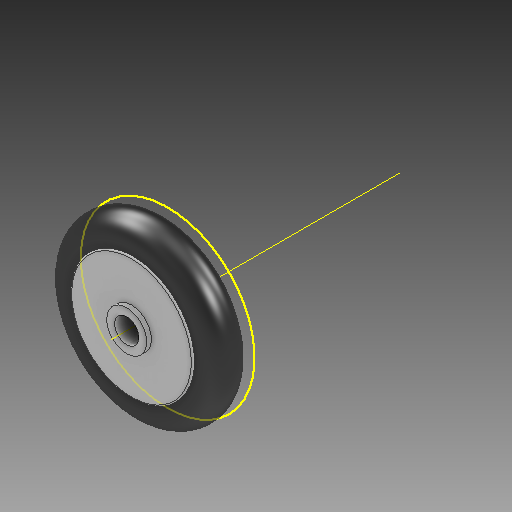
# Autodesk Inventor part: sub_wheel
Saved by Autodesk Inventor 2020 (Build 240168000, 168)
## iProperties
Created: 2024-10-05
Part Number: sub_wheel
Material: Типовые
Document SubType Name: Modeling
Designer: Ivan
Density: 1 g/cm^3
Appearance: По умолчанию
Mass: 0.056422 g
Surface Area: 1.13235 cm^2
Volume: 0.056422 cm^3
Author: Ivan
Autodesk Inventor part; units mm, degrees
ref_plane "YZ Plane" through (0, 0, 0) normal (1, 0, 0) x (0, 1, 0)
ref_plane "XZ Plane" through (0, 0, 0) normal (0, 1, 0) x (-1, 0, 0)
ref_plane "XY Plane" through (0, 0, 0) normal (0, 0, 1) x (1, 0, 0)
sketch "Эскиз1" plane through (0, 0, 0) normal (1, 0, 0) x (0, 1, 0)
  line L0 (0, 0.95) -> (0, -0.95)
  line L1 (0, 0) -> (5, 0) construction
  arc A0 (2.5342, 0.6562) -> (2.5342, -0.6562) centre (2.8973, 0) ccw
  line L2 (2.8973, 0.75) -> (2.8973, -0.75)
  line L3 (2.51, 0.75) -> (0, 0.75)
  line L4 (2.51, -0.75) -> (0, -0.75)
  arc A1 (2.5342, 0.6562) -> (2.51, 0.75) centre (2.51, 0.7) ccw
  arc A2 (2.51, -0.75) -> (2.5342, -0.6562) centre (2.51, -0.7) ccw
  line L5 (0.8367, 0.75) -> (0.8367, 0.95)
  line L6 (0.8367, 0.95) -> (0, 0.95)
  line L7 (0.8367, -0.75) -> (0.8367, -0.95)
  line L8 (0.8367, -0.95) -> (0, -0.95)
  line L9 (0.51, 0.95) -> (0.51, -0.95)
  point P0 (0.51, 0.75)
  point P1 (0.51, -0.75)
  dimension "d0" = 1.9
  dimension "d1" = 5
  dimension "d2" = 1.5
  dimension "d3" = 0.05
  dimension "d4" = 0.8367
  dimension "d5" = 2.51
  dimension "d6" = 0.51
  constraints: 20 end point, 9 point on line, 8 point on circle, 5 tangent, 4 vertical, 3 centre point, 3 horizontal, 3 perpendicular, 2 midpoint, 1 coincident, 1 collinear, 1 equal radius
  measures "d0" distance of L0.start L0.end
  measures "d1" distance of L1.start L1.end
  measures "d2" diameter of A0
  measures "d3" radius of A1
  measures "d4" horizontal distance of L0.start L5.start
  measures "d5" distance of L4.start L4.end
  measures "d6" distance from line of L9 point (0, 0)
revolve "Вращение1" add sketch "Эскиз1" angle 360 about axis through (0, 0, 0.95) along (0, 0, -1) contours L6 L5 L3 L9 | L3 A1 A0 A2 L4 L9 | L4 L7 L8 L9
sketch "Эскиз2" plane through (0, 0, 0) normal (1, 0, 0) x (0, 1, 0)
  arc A0 (-2.5342, -0.6563) -> (-2.5342, 0.6562) centre (-2.8973, 0) ccw projected
  circle A1 centre (-2.8973, 0) radius 0.75
  line L0 (0, 1.33) -> (0, -1.33) projected
  point P0 (0, 0)
  point P1 (-2.5342, 0.6562)
  point P2 (-3.6473, 0)
  dimension "d8" = 1.5
  constraints: 2 point on circle, 1 centre point, 1 coincident
  measures "d8" diameter of A1
revolve "Вращение2" add sketch "Эскиз2" angle 360 about axis through (0, 0, 0) along (0, 0, -1)
sketch "Эскиз3" plane through (0, 0, -0.75) normal (0, 0, -1) x (-1, 0, 0)
  circle A0 centre (0, 0) radius 3.6473 projected
  point P0 (0, 0)
equation "\"d4\" = 0.333333 * d5"
